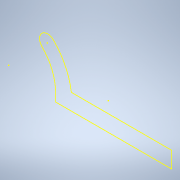
# Autodesk Inventor part: HandleBaseFiller
Saved by Autodesk Inventor 2021 (Build 250183000, 183)
## iProperties
Created: 2021-06-04
Part Number: HandleBaseFiller
Material: Generic
Document SubType Name: Modeling
Designer: teh18
Density: 1 g/cm^3
Appearance: Default
Author: teh18
Autodesk Inventor part; units mm, degrees
ref_plane "YZ Plane" through (0, 0, 0) normal (1, 0, 0) x (0, 1, 0)
ref_plane "XZ Plane" through (0, 0, 0) normal (0, 1, 0) x (-1, 0, 0)
sketch "Sketch1" plane through (0, 0, 0) normal (0, 0, 1) x (1, 0, 0)
  line L0 (19.4574, -8.4881) -> (19.4574, -3.4881) projected
  line L1 (-16.2695, -8.4881) -> (19.4574, -8.4881) projected
  line L2 (-16.2695, -5.9881) -> (-16.2695, -8.4881) projected
  arc A0 (-16.2695, -5.9881) -> (-20.498, 4.2204) centre (-30.7065, -5.9881) ccw projected
  arc A1 (-16.9624, 7.7559) -> (-20.498, 4.2204) centre (-18.7302, 5.9881) ccw projected
  arc A2 (-11.4309, -3.4881) -> (-16.9624, 7.7559) centre (-30.7065, -5.9881) ccw projected
  line L3 (19.4574, -3.4881) -> (-11.4309, -3.4881) projected
  arc A3 (-11.2695, -5.9881) -> (-11.4309, -3.4881) centre (-30.7065, -5.9881) ccw
  line L4 (-11.2695, -5.9881) -> (-11.2695, -8.4881)
  line L5 (-11.2695, -8.4881) -> (19.4574, -8.4881)
  line L6 (19.4574, -8.4881) -> (19.4574, -3.4881)
  line L7 (19.4574, -3.4881) -> (-11.4309, -3.4881)
  line L8 (21.2302, -3.4881) -> (-11.4309, -3.4881) projected
  arc A4 (-11.4309, -3.4881) -> (-16.9624, 7.7559) centre (-30.7065, -5.9881) ccw projected
  arc A5 (-16.9624, 7.7559) -> (-20.498, 4.2204) centre (-18.7302, 5.9881) ccw projected
  arc A6 (-16.2695, -5.9881) -> (-20.498, 4.2204) centre (-30.7065, -5.9881) ccw projected
  line L9 (-16.2695, -5.9881) -> (-16.2695, -8.4881) projected
  line L10 (-16.2695, -8.4881) -> (21.2302, -8.4881) projected
  line L11 (21.2302, -25.9881) -> (21.2302, -8.4881) projected
  line L12 (21.2302, -25.9881) -> (-52.4119, -25.9881) projected
  line L13 (-52.4119, -25.9881) -> (-52.4119, 14.0119) projected
  line L14 (21.2302, 14.0119) -> (-52.4119, 14.0119) projected
  line L15 (21.2302, -3.4881) -> (21.2302, 14.0119) projected
  circle A7 centre (-30.7065, -5.9881) radius 9.525 projected
  line L16 (19.4574, -3.4881) -> (21.2302, -3.4881)
  line L17 (21.2302, -3.4881) -> (21.2302, -8.4881)
  line L18 (21.2302, -8.4881) -> (19.4574, -8.4881)
  line L19 (19.4574, -8.4881) -> (19.4574, -3.4881)
  point P0 (0, 0)
  constraints: 16 end point, 4 equal length, 2 horizontal, 2 perpendicular, 2 point on circle, 1 centre point, 1 coincident, 1 point on line
ref_plane "Work Plane1" through (-44.9119, -25.9881, 5) normal (0, 0, 1) x (1, 0, 0)
extrude "Extrusion1" add sketch "Sketch1" along normal up to surface (5 mm away) contours L1 L4 A3 L3 L0 | L0 L8 L17 L10
sketch "Sketch2" plane through (-11.4309, -3.4881, 0) normal (0, 1, 0) x (1, 0, 0)
  line L0 (32.6611, -25) -> (-40.9809, -25) projected
  line L1 (-40.9809, -25) -> (-40.9809, -5) projected
  line L2 (-40.9809, -5) -> (32.6611, -5) projected
  arc A0 (32.6611, -5) -> (-38.4667, -1.5) centre (-3.4809, -15) ccw projected
  line L3 (-38.4667, -1.5) -> (-43.4667, -1.5) projected
  line L4 (-43.4667, -1.5) -> (-47.1748, -15) projected
  line L5 (-47.1748, -15) -> (-43.4667, -28.5) projected
  line L6 (-43.4667, -28.5) -> (-38.4667, -28.5) projected
  arc A1 (-38.4667, -28.5) -> (32.6611, -25) centre (-3.4809, -15) ccw projected
  line L7 (32.6611, 0) -> (0, 0) projected
  line L8 (32.6611, 0) -> (32.6611, -5) projected
  point P0 (11.4309, 0)
  point P1 (30.8884, 0)
extrude "Extrusion2" cut sketch "Sketch2" against normal through all contours A0 L7 L8
body "Solid1"
